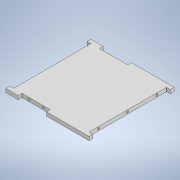
# Autodesk Inventor part: baza
Saved by Autodesk Inventor 2020 (Build 240168000, 168)
## iProperties
Created: 2020-08-17
Part Number: baza
Material: Generic
Document SubType Name: Modeling
Designer: Hesekiel
Density: 1 g/cm^3
Appearance: Default
Author: Hesekiel
Autodesk Inventor part; units mm, degrees
ref_plane "YZ Plane" through (0, 0, 0) normal (1, 0, 0) x (0, 1, 0)
ref_plane "XZ Plane" through (0, 0, 0) normal (0, 1, 0) x (-1, 0, 0)
ref_plane "XY Plane" through (0, 0, 0) normal (0, 0, 1) x (1, 0, 0)
sketch "Sketch1" plane through (0, 0, 0) normal (0, 1, 0) x (-1, 0, 0)
  line L0 (-50, 112.5) -> (50, 112.5)
  line L1 (50, 112.5) -> (50, -112.5)
  line L2 (50, -112.5) -> (-50, -112.5)
  line L3 (-50, -112.5) -> (-50, 112.5)
  line L4 (-50, 112.5) -> (50, -112.5) construction
  line L5 (50, 112.5) -> (-50, -112.5) construction
  line L6 (-37.5, -102.5) -> (37.5, -102.5)
  line L7 (37.5, -102.5) -> (37.5, 102.5)
  line L8 (37.5, 102.5) -> (-37.5, 102.5)
  line L9 (-37.5, 102.5) -> (-37.5, -102.5)
  line L10 (-37.5, -102.5) -> (37.5, 102.5) construction
  line L11 (37.5, -102.5) -> (-37.5, 102.5) construction
  line L12 (37.5, 112.5) -> (37.5, -112.5)
  line L13 (-37.5, 112.5) -> (-37.5, -112.5)
  line L14 (-50, -112.5) -> (-150, -112.5)
  line L15 (-150, 112.5) -> (-50, 112.5)
  line L16 (-50, 112.5) -> (-50, -112.5)
  line L17 (-150, -112.5) -> (-140, -112.5)
  line L18 (-140, -112.5) -> (-140, 112.5)
  line L19 (-150, -112.5) -> (-150, -102.5)
  line L20 (-150, -102.5) -> (-140, -102.5)
  line L21 (-140, 112.5) -> (-140, 102.5)
  line L22 (-140, 102.5) -> (-150, 102.5)
  line L23 (50, 112.5) -> (70, 112.5)
  line L24 (70, -112.5) -> (50, -112.5)
  line L25 (50, -112.5) -> (50, 112.5)
  line L26 (70, -112.5) -> (70, -102.5)
  line L27 (70, 112.5) -> (70, 102.5)
  line L28 (70, -102.5) -> (60, -102.5)
  line L29 (60, -102.5) -> (60, 102.5)
  line L30 (60, 102.5) -> (70, 102.5)
  line L31 (-150, 102.5) -> (-150, 112.5)
  point P0 (0, 0)
  dimension "d0" = 100
  dimension "d2" = 75
  dimension "d3" = 205
  dimension "d49" = 100
  dimension "d50" = 10
  dimension "d51" = 10
  dimension "d52" = 10
  constraints: 64 end point, 11 point on line, 7 parallel, 5 horizontal, 5 perpendicular, 4 midpoint, 1 vertical
  measures "d0" distance of L1.end L2.end
  measures "d2" distance of L8.end L7.end
  measures "d3" distance of L7.end L6.end
  measures "d49" distance of L15.start L15.end
  measures "d50" distance of L14.end L17.end
  measures "d51" distance of L14.end L19.end
  measures "d52" distance of L18.end L21.end
extrude "Extrusion1" add sketch "Sketch1" along normal blind 10 contours L0 L13 L9 L2 L3 | L3 L14 L18 L15 | L18 L22 L31 L15 | L0 L1 L2 L12 L7 | L8 L7 L6 L9 | L14 L19 L20 L18 | L23 L27 L30 L29 L28 L26 L24 L1
sketch "Sketch2" plane through (-37.5, 0, 102.5) normal (0, 0, 1) x (1, 0, 0)
  line L0 (0, 0) -> (75, 0) projected
  line L1 (75, 0) -> (75, 10) projected
  line L2 (0, 10) -> (75, 10) projected
  line L3 (0, 0) -> (0, 10) projected
  line L4 (37.5, 0) -> (37.5, 10)
  line L5 (75, 10) -> (0, 10) projected
  line L6 (37.5, 5) -> (0, 5)
  line L7 (0, 0) -> (0, 10) projected
  line L8 (37.5, 5) -> (75, 5)
  line L9 (75, 0) -> (75, 10) projected
  circle A0 centre (18.75, 5) radius 3
  circle A1 centre (56.25, 5) radius 3
  dimension "d6" = 6
  dimension "d7" = 6
  constraints: 6 end point, 6 midpoint, 2 centre point
  measures "d6" diameter of A0
  measures "d7" diameter of A1
extrude "Extrusion2" cut sketch "Sketch2" against normal blind 20 contours A0 L6 | L6 A0 | A1 L8 | L8 A1
thread "Thread1" size "M6x1" class "6H" standard "ANSI Metric M Profile" full length
thread "Thread2" size "M6x1" class "6H" standard "ANSI Metric M Profile" full length
sketch "Sketch3" plane through (37.5, 0, -102.5) normal (0, 0, -1) x (-1, 0, 0)
  circle A0 centre (18.75, 5) radius 3 projected
  circle A1 centre (56.25, 5) radius 3 projected
  point P0 (37.5, 0)
extrude "Extrusion3" cut sketch "Sketch3" against normal blind 20
thread "Thread3" size "M6x1" class "6H" standard "ANSI Metric M Profile" full length
thread "Thread4" size "M6x1" class "6H" standard "ANSI Metric M Profile" full length
sketch "Sketch4" plane through (-18.75, 5, 82.5) normal (0, 0, 1) x (1, 0, 0)
  point P0 (0, 0)
hole "Hole1" at (-18.75, 5, 82.5) direction (0, 0, -1) diameter 4.917 depth 6 tip angle 120 thread size "M6x1" class "6H" standard "ISO Metric profile"
sketch "Sketch5" plane through (18.75, 5, 82.5) normal (0, 0, 1) x (1, 0, 0)
  point P0 (0, 0)
hole "Hole3" at (18.75, 5, 82.5) direction (0, 0, -1) diameter 4.917 depth 6 tip angle 120 thread size "M6x1" class "6H" standard "ISO Metric profile"
sketch "Sketch6" plane through (18.75, 5, -82.5) normal (0, 0, -1) x (-1, 0, 0)
  point P0 (0, 0)
hole "Hole5" at (18.75, 5, -82.5) direction (0, 0, 1) diameter 4.917 depth 6 tip angle 120 thread size "M6x1" class "6H" standard "ISO Metric profile"
sketch "Sketch7" plane through (-18.75, 5, -82.5) normal (0, 0, -1) x (-1, 0, 0)
  point P0 (0, 0)
hole "Hole7" at (-18.75, 5, -82.5) direction (0, 0, 1) diameter 4.917 depth 6 tip angle 120 thread size "M6x1" class "6H" standard "ISO Metric profile"
fillet "Fillet1" radius 1 6 edges at (-37.5, 5, 102.5) (37.5, 5, 102.5) (-37.5, 5, -102.5) (37.5, 5, -102.5) (140, 5, -102.5) (140, 5, 102.5)
sketch "Sketch8" plane through (140, 0, 101.5) normal (1, 0, 0) x (0, 0, -1)
  line L0 (0, 0) -> (0, 10) projected
  line L1 (0, 0) -> (203, 0) projected
  line L2 (203, 10) -> (203, 0) projected
  line L3 (0, 10) -> (203, 10) projected
  line L4 (214, 10) -> (-11, 10) projected
  circle A0 centre (100.5, 5) radius 3
  line L5 (203, 10) -> (203, 0) projected
  line L6 (178, 2.5415) -> (178, 7.4585) projected
  circle A1 centre (178, 5) radius 3
  circle A2 centre (24, 5) radius 3
  point P0 (101.5, 0)
  dimension "d54" = 6
  dimension "d57" = 6
  dimension "d59" = 6
  constraints: 3 centre point, 1 midpoint
  measures "d54" diameter of A0
  measures "d57" diameter of A1
  measures "d59" diameter of A2
extrude "Extrusion4" cut sketch "Sketch8" against normal blind 30 contours A0 | A1 | A2
thread "Thread5" size "M6x1" class "6H" standard "ANSI Metric M Profile" full length
thread "Thread6" size "M6x1" class "6H" standard "ANSI Metric M Profile" full length
thread "Thread7" size "M6x1" class "6H" standard "ANSI Metric M Profile" full length
sketch "Sketch9" plane through (110, 5, 77.5) normal (1, 0, 0) x (0, 0, -1)
  point P0 (-0.375, 0)
hole "Hole9" at (110, 5, 77.875) direction (-1, 0, 0) diameter 4.917 depth 6 tip angle 120 thread size "M6x1" class "6H" standard "ISO Metric profile"
sketch "Sketch10" plane through (110, 5, 1) normal (1, 0, 0) x (0, 0, -1)
  point P0 (0, 0)
hole "Hole11" at (110, 5, 1) direction (-1, 0, 0) diameter 4.917 depth 6 tip angle 120 thread size "M6x1" class "6H" standard "ISO Metric profile"
sketch "Sketch11" plane through (110, 5, -76.5) normal (1, 0, 0) x (0, 0, -1)
  point P0 (0.375, 0)
hole "Hole13" at (110, 5, -76.875) direction (-1, 0, 0) diameter 4.917 depth 6 tip angle 120 thread size "M6x1" class "6H" standard "ISO Metric profile"
sketch "Sketch12" plane through (-60, 0, -102.5) normal (-1, 0, 0) x (0, 0, 1)
  circle A0 centre (26, 5) radius 3 projected
  circle A1 centre (103.5, 5) radius 3 projected
  circle A2 centre (180, 5) radius 3 projected
  line L0 (204, 0) -> (204, 10) projected
  line L1 (204, 0) -> (1, 0) projected
  line L2 (1, 10) -> (1, 0) projected
  line L3 (204, 10) -> (1, 10) projected
  point P0 (102.5, 0)
extrude "Extrusion5" cut sketch "Sketch12" against normal blind 30 contours A0 | A1 | A2
thread "Thread8" size "M6x1" class "6H" standard "ANSI Metric M Profile" full length
thread "Thread9" size "M6x1" class "6H" standard "ANSI Metric M Profile" full length
thread "Thread10" size "M6x1" class "6H" standard "ANSI Metric M Profile" full length
body "Solid1"
